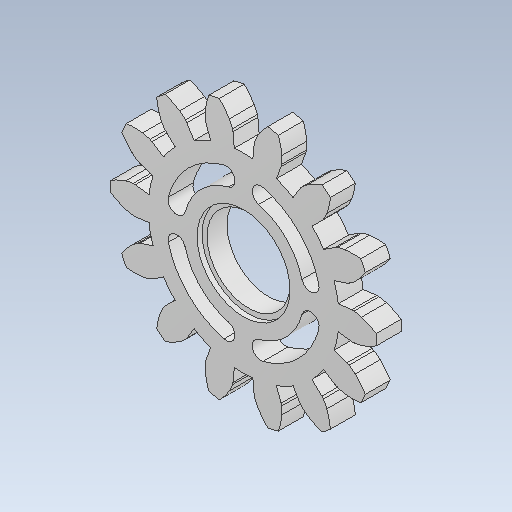
# Autodesk Inventor part: ｍ2歯数14ギアd10
Saved by Autodesk Inventor 2020.2 (Build 242310000, 310)
## iProperties
Created: 2020-03-09
Part Number: ｍ2歯数14ギアd10
Material: アルミニウム 2014-T4
Document SubType Name: Modeling
Designer: aoyam
Density: 2.8 g/cm^3
Appearance: サテン
Mass: 4.28588 g
Surface Area: 16.7705 cm^2
Volume: 1.53067 cm^3
Author: aoyam
Autodesk Inventor part; units mm, degrees
ref_plane "YZ Plane" through (0, 0, 0) normal (1, 0, 0) x (0, 1, 0)
ref_plane "XZ Plane" through (0, 0, 0) normal (0, 1, 0) x (-1, 0, 0)
ref_plane "XY Plane" through (0, 0, 0) normal (0, 0, 1) x (1, 0, 0)
sketch "スケッチ1" plane through (0, 0, 0) normal (0, 0, 1) x (1, 0, 0)
  arc A0 (3.027306, 14.807993) -> (2.963603, 14.540405) centre (4.457622, 14.32611) ccw
  arc A1 (3.408783, 15.648143) -> (3.027306, 14.807993) centre (7.00507, 13.50854) ccw
  arc A2 (4.613453, 17.176768) -> (3.408783, 15.648143) centre (9.745262, 11.893521) ccw
  arc A3 (0.407664, 14.540405) -> (0.343961, 14.807993) centre (-1.086355, 14.32611) ccw
  arc A4 (0.343961, 14.807993) -> (-0.037516, 15.648143) centre (-3.633803, 13.50854) ccw
  arc A5 (-0.037516, 15.648143) -> (-1.242186, 17.176768) centre (-6.373995, 11.893521) ccw
  arc A6 (2.802766, 12.892539) -> (0.568501, 12.892539) centre (1.685634, 1.446928) ccw
  arc A7 (-1.242186, 17.176768) -> (-2.501414, 16.889357) centre (1.685634, 1.446928) ccw
  line L0 (2.802766, 12.892539) -> (2.963603, 14.540405)
  line L1 (0.568501, 12.892539) -> (0.407664, 14.540405)
  arc A8 (-6.028546, 13.494134) -> (-7.777163, 14.34869) centre (-10.108448, 7.362041) ccw
  arc A9 (-7.777163, 14.34869) -> (-8.786985, 13.543384) centre (1.685634, 1.446928) ccw
  arc A10 (-5.320321, 12.902702) -> (-6.028546, 13.494134) centre (-8.340351, 10.006048) ccw
  arc A11 (-5.146824, 12.689253) -> (-5.320321, 12.902702) centre (-6.39991, 11.847949) ccw
  line L2 (-4.286932, 11.274361) -> (-5.146824, 12.689253)
  arc A12 (-2.90271, 14.066962) -> (-2.844002, 13.798233) centre (-1.404959, 14.253391) ccw
  arc A13 (-2.923539, 14.989427) -> (-2.90271, 14.066962) centre (1.244943, 14.622082) ccw
  arc A14 (-2.501414, 16.889357) -> (-2.923539, 14.989427) centre (4.414501, 14.355925) ccw
  line L3 (-2.27393, 12.243772) -> (-2.844002, 13.798233)
  arc A15 (-2.27393, 12.243772) -> (-4.286932, 11.274361) centre (1.685634, 1.446928) ccw
  arc A16 (-10.491689, 8.954028) -> (-12.437917, 8.965261) centre (-11.506938, 1.659001) ccw
  arc A17 (-12.437917, 8.965261) -> (-12.998325, 7.80156) centre (1.685634, 1.446928) ccw
  arc A18 (-9.596987, 8.728454) -> (-10.491689, 8.954028) centre (-11.061129, 4.808317) ccw
  arc A19 (-9.34806, 8.61142) -> (-9.596987, 8.728454) centre (-10.112023, 7.309739) ccw
  line L4 (-7.959426, 7.70974) -> (-9.34806, 8.61142)
  arc A20 (-7.923949, 10.826378) -> (-7.754458, 10.609734) centre (-6.65541, 11.644194) ccw
  arc A21 (-8.342958, 11.648453) -> (-7.923949, 10.826378) centre (-4.4279, 13.126123) ccw
  arc A22 (-8.786985, 13.543384) -> (-8.342958, 11.648453) centre (-1.456746, 14.261543) ccw
  line L5 (-6.566385, 9.456558) -> (-7.754458, 10.609734)
  arc A23 (-6.566385, 9.456558) -> (-7.959426, 7.70974) centre (1.685634, 1.446928) ccw
  arc A24 (-12.542964, 2.927049) -> (-14.301328, 2.092733) centre (-10.292478, -4.086043) ccw
  arc A25 (-14.301328, 2.092733) -> (-14.301328, 0.801122) centre (1.685634, 1.446928) ccw
  arc A26 (-11.638992, 3.11201) -> (-12.542964, 2.927049) centre (-11.257255, -1.055178) ccw
  arc A27 (-11.363938, 3.114572) -> (-11.638992, 3.11201) centre (-11.487466, 1.610326) ccw
  line L6 (-9.721598, 2.904692) -> (-11.363938, 3.114572)
  arc A28 (-11.041892, 5.728079) -> (-10.795188, 5.606429) centre (-10.253815, 7.015304) ccw
  arc A29 (-11.776091, 6.286941) -> (-11.041892, 5.728079) centre (-8.889883, 9.316956) ccw
  arc A30 (-12.998325, 7.80156) -> (-11.776091, 6.286941) centre (-6.705606, 11.62907) ccw
  line L7 (-9.224427, 5.082939) -> (-10.795188, 5.606429)
  arc A31 (-9.224427, 5.082939) -> (-9.721598, 2.904692) centre (1.685634, 1.446928) ccw
  arc A32 (-11.776091, -3.393086) -> (-12.998325, -4.907705) centre (-6.705606, -8.735215) ccw
  arc A33 (-12.998325, -4.907705) -> (-12.437917, -6.071406) centre (1.685634, 1.446928) ccw
  arc A34 (-11.041892, -2.834223) -> (-11.776091, -3.393086) centre (-8.889883, -6.423101) ccw
  arc A35 (-10.795188, -2.712574) -> (-11.041892, -2.834223) centre (-10.253815, -4.121449) ccw
  line L8 (-9.224427, -2.189084) -> (-10.795188, -2.712574)
  arc A36 (-11.638992, -0.218155) -> (-11.363938, -0.220717) centre (-11.487466, 1.283529) ccw
  arc A37 (-12.542964, -0.033194) -> (-11.638992, -0.218155) centre (-11.257255, 3.949033) ccw
  arc A38 (-14.301328, 0.801122) -> (-12.542964, -0.033194) centre (-10.292478, 6.979898) ccw
  line L9 (-9.721598, -0.010837) -> (-11.363938, -0.220717)
  arc A39 (-9.721598, -0.010837) -> (-9.224427, -2.189084) centre (1.685634, 1.446928) ccw
  arc A40 (-8.342958, -8.754598) -> (-8.786985, -10.649529) centre (-1.456746, -11.367688) ccw
  arc A41 (-8.786985, -10.649529) -> (-7.777163, -11.454835) centre (1.685634, 1.446928) ccw
  arc A42 (-7.923949, -7.932523) -> (-8.342958, -8.754598) centre (-4.4279, -10.232268) ccw
  arc A43 (-7.754458, -7.715879) -> (-7.923949, -7.932523) centre (-6.65541, -8.750339) ccw
  line L10 (-6.566385, -6.562703) -> (-7.754458, -7.715879)
  arc A44 (-9.596987, -5.834599) -> (-9.34806, -5.717565) centre (-10.112023, -4.415883) ccw
  arc A45 (-10.491689, -6.060173) -> (-9.596987, -5.834599) centre (-11.061129, -1.914462) ccw
  arc A46 (-12.437917, -6.071406) -> (-10.491689, -6.060173) centre (-11.506938, 1.234854) ccw
  line L11 (-7.959426, -4.815885) -> (-9.34806, -5.717565)
  arc A47 (-7.959426, -4.815885) -> (-6.566385, -6.562703) centre (1.685634, 1.446928) ccw
  arc A48 (-2.923539, -12.095572) -> (-2.501414, -13.995502) centre (4.414501, -11.462069) ccw
  arc A49 (-2.501414, -13.995502) -> (-1.242186, -14.282913) centre (1.685634, 1.446928) ccw
  arc A50 (-2.90271, -11.173107) -> (-2.923539, -12.095572) centre (1.244943, -11.728227) ccw
  arc A51 (-2.844002, -10.904378) -> (-2.90271, -11.173107) centre (-1.404959, -11.359536) ccw
  line L12 (-2.27393, -9.349917) -> (-2.844002, -10.904378)
  arc A52 (-5.320321, -10.008847) -> (-5.146824, -9.795398) centre (-6.39991, -8.954094) ccw
  arc A53 (-6.028546, -10.600279) -> (-5.320321, -10.008847) centre (-8.340351, -7.112193) ccw
  arc A54 (-7.777163, -11.454835) -> (-6.028546, -10.600279) centre (-10.108448, -4.468186) ccw
  line L13 (-4.286932, -8.380506) -> (-5.146824, -9.795398)
  arc A55 (-4.286932, -8.380506) -> (-2.27393, -9.349917) centre (1.685634, 1.446928) ccw
  arc A56 (3.408783, -12.754288) -> (4.613453, -14.282913) centre (9.745262, -8.999666) ccw
  arc A57 (4.613453, -14.282913) -> (5.872681, -13.995502) centre (1.685634, 1.446928) ccw
  arc A58 (3.027306, -11.914138) -> (3.408783, -12.754288) centre (7.00507, -10.614685) ccw
  arc A59 (2.963603, -11.64655) -> (3.027306, -11.914138) centre (4.457622, -11.432255) ccw
  line L14 (2.802766, -9.998684) -> (2.963603, -11.64655)
  arc A60 (0.343961, -11.914138) -> (0.407664, -11.64655) centre (-1.086355, -11.432255) ccw
  arc A61 (-0.037516, -12.754288) -> (0.343961, -11.914138) centre (-3.633803, -10.614685) ccw
  arc A62 (-1.242186, -14.282913) -> (-0.037516, -12.754288) centre (-6.373995, -8.999666) ccw
  line L15 (0.568501, -9.998684) -> (0.407664, -11.64655)
  arc A63 (0.568501, -9.998684) -> (2.802766, -9.998684) centre (1.685634, 1.446928) ccw
  arc A64 (9.399814, -10.600279) -> (11.14843, -11.454835) centre (13.479715, -4.468186) ccw
  arc A65 (11.14843, -11.454835) -> (12.158252, -10.649529) centre (1.685634, 1.446928) ccw
  arc A66 (8.691588, -10.008847) -> (9.399814, -10.600279) centre (11.711618, -7.112193) ccw
  arc A67 (8.518091, -9.795398) -> (8.691588, -10.008847) centre (9.771177, -8.954094) ccw
  line L16 (7.658199, -8.380506) -> (8.518091, -9.795398)
  arc A68 (6.273977, -11.173107) -> (6.21527, -10.904378) centre (4.776226, -11.359536) ccw
  arc A69 (6.294806, -12.095572) -> (6.273977, -11.173107) centre (2.126324, -11.728227) ccw
  arc A70 (5.872681, -13.995502) -> (6.294806, -12.095572) centre (-1.043234, -11.462069) ccw
  line L17 (5.645197, -9.349917) -> (6.21527, -10.904378)
  arc A71 (5.645197, -9.349917) -> (7.658199, -8.380506) centre (1.685634, 1.446928) ccw
  arc A72 (13.862957, -6.060173) -> (15.809184, -6.071406) centre (14.878205, 1.234854) ccw
  arc A73 (15.809184, -6.071406) -> (16.369593, -4.907705) centre (1.685634, 1.446928) ccw
  arc A74 (12.968255, -5.834599) -> (13.862957, -6.060173) centre (14.432396, -1.914462) ccw
  arc A75 (12.719327, -5.717565) -> (12.968255, -5.834599) centre (13.48329, -4.415883) ccw
  line L18 (11.330693, -4.815885) -> (12.719327, -5.717565)
  arc A76 (11.295216, -7.932523) -> (11.125725, -7.715879) centre (10.026677, -8.750339) ccw
  arc A77 (11.714225, -8.754598) -> (11.295216, -7.932523) centre (7.799167, -10.232268) ccw
  arc A78 (12.158252, -10.649529) -> (11.714225, -8.754598) centre (4.828013, -11.367688) ccw
  line L19 (9.937652, -6.562703) -> (11.125725, -7.715879)
  arc A79 (9.937652, -6.562703) -> (11.330693, -4.815885) centre (1.685634, 1.446928) ccw
  arc A80 (15.914231, -0.033194) -> (17.672595, 0.801122) centre (13.663745, 6.979898) ccw
  arc A81 (17.672595, 0.801122) -> (17.672595, 2.092733) centre (1.685634, 1.446928) ccw
  arc A82 (15.01026, -0.218155) -> (15.914231, -0.033194) centre (14.628522, 3.949033) ccw
  arc A83 (14.735205, -0.220717) -> (15.01026, -0.218155) centre (14.858733, 1.283529) ccw
  line L20 (13.092865, -0.010837) -> (14.735205, -0.220717)
  arc A84 (14.413159, -2.834223) -> (14.166455, -2.712574) centre (13.625082, -4.121449) ccw
  arc A85 (15.147358, -3.393086) -> (14.413159, -2.834223) centre (12.26115, -6.423101) ccw
  arc A86 (16.369593, -4.907705) -> (15.147358, -3.393086) centre (10.076873, -8.735215) ccw
  line L21 (12.595694, -2.189084) -> (14.166455, -2.712574)
  arc A87 (12.595694, -2.189084) -> (13.092865, -0.010837) centre (1.685634, 1.446928) ccw
  arc A88 (15.147358, 6.286941) -> (16.369593, 7.80156) centre (10.076873, 11.62907) ccw
  arc A89 (16.369593, 7.80156) -> (15.809184, 8.965261) centre (1.685634, 1.446928) ccw
  arc A90 (14.413159, 5.728079) -> (15.147358, 6.286941) centre (12.26115, 9.316956) ccw
  arc A91 (14.166455, 5.606429) -> (14.413159, 5.728079) centre (13.625082, 7.015304) ccw
  line L22 (12.595694, 5.082939) -> (14.166455, 5.606429)
  arc A92 (15.01026, 3.11201) -> (14.735205, 3.114572) centre (14.858733, 1.610326) ccw
  arc A93 (15.914231, 2.927049) -> (15.01026, 3.11201) centre (14.628522, -1.055178) ccw
  arc A94 (17.672595, 2.092733) -> (15.914231, 2.927049) centre (13.663745, -4.086043) ccw
  line L23 (13.092865, 2.904692) -> (14.735205, 3.114572)
  arc A95 (13.092865, 2.904692) -> (12.595694, 5.082939) centre (1.685634, 1.446928) ccw
  arc A96 (11.714225, 11.648453) -> (12.158252, 13.543384) centre (4.828013, 14.261543) ccw
  arc A97 (12.158252, 13.543384) -> (11.14843, 14.34869) centre (1.685634, 1.446928) ccw
  arc A98 (11.295216, 10.826378) -> (11.714225, 11.648453) centre (7.799167, 13.126123) ccw
  arc A99 (11.125725, 10.609734) -> (11.295216, 10.826378) centre (10.026677, 11.644194) ccw
  line L24 (9.937652, 9.456558) -> (11.125725, 10.609734)
  arc A100 (12.968255, 8.728454) -> (12.719327, 8.61142) centre (13.48329, 7.309739) ccw
  arc A101 (13.862957, 8.954028) -> (12.968255, 8.728454) centre (14.432396, 4.808317) ccw
  arc A102 (15.809184, 8.965261) -> (13.862957, 8.954028) centre (14.878205, 1.659001) ccw
  line L25 (11.330693, 7.70974) -> (12.719327, 8.61142)
  arc A103 (11.330693, 7.70974) -> (9.937652, 9.456558) centre (1.685634, 1.446928) ccw
  arc A104 (6.294806, 14.989427) -> (5.872681, 16.889357) centre (-1.043234, 14.355925) ccw
  arc A105 (5.872681, 16.889357) -> (4.613453, 17.176768) centre (1.685634, 1.446928) ccw
  arc A106 (6.273977, 14.066962) -> (6.294806, 14.989427) centre (2.126324, 14.622082) ccw
  arc A107 (6.21527, 13.798233) -> (6.273977, 14.066962) centre (4.776226, 14.253391) ccw
  line L26 (5.645197, 12.243772) -> (6.21527, 13.798233)
  arc A108 (8.691588, 12.902702) -> (8.518091, 12.689253) centre (9.771177, 11.847949) ccw
  arc A109 (9.399814, 13.494134) -> (8.691588, 12.902702) centre (11.711618, 10.006048) ccw
  arc A110 (11.14843, 14.34869) -> (9.399814, 13.494134) centre (13.479715, 7.362041) ccw
  line L27 (7.658199, 11.274361) -> (8.518091, 12.689253)
  arc A111 (7.658199, 11.274361) -> (5.645197, 12.243772) centre (1.685634, 1.446928) ccw
  circle A112 centre (1.685634, 1.446928) radius 5
  circle A113 centre (1.685634, 1.446928) radius 11.5
  circle A114 centre (1.685634, 1.446928) radius 9.375343
  circle A115 centre (1.685634, 1.446928) radius 7.275343
  line L28 (6.685634, 1.446928) -> (-7.68971, 1.446928)
  circle A116 centre (-6.373995, 3.533487) radius 1.05
  circle A117 centre (-6.373995, -0.639632) radius 1.05
  circle A118 centre (-0.400926, -6.612701) radius 1.05
  circle A119 centre (3.772193, -6.612701) radius 1.05
  circle A120 centre (9.745262, -0.639632) radius 1.05
  circle A121 centre (9.745262, 3.533487) radius 1.05
  circle A122 centre (3.772193, 9.506556) radius 1.05
  circle A123 centre (-0.400926, 9.506556) radius 1.05
  point P0 (0, 0)
  point P1 (6.21527, 13.798233)
  point P2 (6.273977, 14.066962)
  point P3 (6.294806, 14.989427)
  point P4 (5.872681, 16.889357)
  point P5 (4.613453, 17.176768)
  point P6 (3.408783, 15.648143)
  point P7 (3.027306, 14.807993)
  point P8 (0.343961, 14.807993)
  point P9 (-0.037516, 15.648143)
  point P10 (-1.242186, 17.176768)
  point P11 (-2.501414, 16.889357)
  point P12 (-2.923539, 14.989427)
  point P13 (-2.90271, 14.066962)
  point P14 (-2.844002, 13.798233)
  point P15 (-2.27393, 12.243772)
  point P16 (-4.286932, 11.274361)
  point P17 (-5.146824, 12.689253)
  point P18 (-5.320321, 12.902702)
  point P19 (-6.028546, 13.494134)
  point P20 (-7.777163, 14.34869)
  point P21 (-8.786985, 13.543384)
  point P22 (-8.342958, 11.648453)
  point P23 (-7.754458, 10.609734)
  point P24 (-6.566385, 9.456558)
  point P25 (-7.959426, 7.70974)
  point P26 (-9.34806, 8.61142)
  point P27 (-9.596987, 8.728454)
  point P28 (-10.491689, 8.954028)
  point P29 (-12.437917, 8.965261)
  point P30 (-12.998325, 7.80156)
  point P31 (-11.776091, 6.286941)
  point P32 (-11.041892, 5.728079)
  point P33 (-10.795188, 5.606429)
  point P34 (-11.363938, 3.114572)
  point P35 (-11.638992, 3.11201)
  point P36 (-12.542964, 2.927049)
  point P37 (-14.301328, 2.092733)
  point P38 (-14.301328, 0.801122)
  point P39 (-12.542964, -0.033194)
  point P40 (-11.638992, -0.218155)
  point P41 (-11.363938, -0.220717)
  point P42 (-9.721598, -0.010837)
  point P43 (-10.795188, -2.712574)
  point P44 (-11.041892, -2.834223)
  point P45 (-11.776091, -3.393086)
  point P46 (-12.998325, -4.907705)
  point P47 (-12.437917, -6.071406)
  point P48 (-10.491689, -6.060173)
  point P49 (-9.596987, -5.834599)
  point P50 (-9.34806, -5.717565)
  point P51 (-7.923949, -7.932523)
  point P52 (-8.342958, -8.754598)
  point P53 (-8.786985, -10.649529)
  point P54 (-7.777163, -11.454835)
  point P55 (-6.028546, -10.600279)
  point P56 (-5.320321, -10.008847)
  point P57 (-5.146824, -9.795398)
  point P58 (-4.286932, -8.380506)
  point P59 (-2.844002, -10.904378)
  point P60 (-2.90271, -11.173107)
  point P61 (-2.923539, -12.095572)
  point P62 (-2.501414, -13.995502)
  point P63 (-1.242186, -14.282913)
  point P64 (-0.037516, -12.754288)
  point P65 (0.343961, -11.914138)
  point P66 (0.568501, -9.998684)
  point P67 (2.802766, -9.998684)
  point P68 (3.027306, -11.914138)
  point P69 (3.408783, -12.754288)
  point P70 (4.613453, -14.282913)
  point P71 (5.872681, -13.995502)
  point P72 (6.294806, -12.095572)
  point P73 (6.273977, -11.173107)
  point P74 (5.645197, -9.349917)
  point P75 (7.658199, -8.380506)
  point P76 (8.691588, -10.008847)
  point P77 (9.399814, -10.600279)
  point P78 (11.14843, -11.454835)
  point P79 (12.158252, -10.649529)
  point P80 (11.295216, -7.932523)
  point P81 (11.125725, -7.715879)
  point P82 (12.719327, -5.717565)
  point P83 (12.968255, -5.834599)
  point P84 (13.862957, -6.060173)
  point P85 (15.809184, -6.071406)
  point P86 (16.369593, -4.907705)
  point P87 (15.147358, -3.393086)
  point P88 (14.413159, -2.834223)
  point P89 (14.166455, -2.712574)
  point P90 (14.735205, -0.220717)
  point P91 (15.01026, -0.218155)
  point P92 (15.914231, -0.033194)
  point P93 (17.672595, 0.801122)
  point P94 (17.672595, 2.092733)
  point P95 (15.914231, 2.927049)
  point P96 (15.01026, 3.11201)
  point P97 (13.092865, 2.904692)
  point P98 (12.595694, 5.082939)
  point P99 (14.413159, 5.728079)
  point P100 (15.147358, 6.286941)
  point P101 (16.369593, 7.80156)
  point P102 (15.809184, 8.965261)
  point P103 (13.862957, 8.954028)
  point P104 (12.968255, 8.728454)
  point P105 (11.330693, 7.70974)
  point P106 (9.937652, 9.456558)
  point P107 (11.295216, 10.826378)
  point P108 (11.714225, 11.648453)
  point P109 (12.158252, 13.543384)
  point P110 (11.14843, 14.34869)
  point P111 (9.399814, 13.494134)
  point P112 (8.518091, 12.689253)
  point P113 (-5.357507, 3.270328)
  point P114 (-7.390483, 3.796646)
  point P115 (-0.664085, 10.523044)
  point P116 (-0.137767, 8.490068)
  point P117 (4.035352, -7.629189)
  point P118 (3.509034, -5.596213)
  point P119 (8.728774, -0.376473)
  point P120 (10.76175, -0.902791)
  point P121 (10.76175, 3.796646)
  point P122 (8.728774, 3.270328)
  point P123 (3.509034, 8.490068)
  point P124 (4.035352, 10.523044)
  point P125 (-7.390483, -0.902791)
  point P126 (-5.357507, -0.376473)
  point P127 (-0.137767, -5.596213)
  point P128 (-0.664085, -7.629189)
  dimension "d4" = 10
  dimension "d2" = 360
  dimension "d21" = 2.12466
  dimension "d22" = 2.27534
  dimension "d24" = 2.1
  dimension "d27" = 360
  constraints: 224 point on circle, 122 centre point, 58 end point, 3 coincident, 1 horizontal alignment, 1 point on line, 1 symmetric about line, 1 tangent, 594 other
  measures "d24" diameter of A116
sketch "スケッチ1 outline for 押し出し1" plane through (0, 0, 0) normal (0, 0, 1) x (1, 0, 0)
  arc A0 (11.295216, -7.932523) -> (11.125725, -7.715879) centre (10.026677, -8.750339) ccw
  arc A1 (11.714225, -8.754598) -> (11.295216, -7.932523) centre (7.799167, -10.232268) ccw
  line L0 (11.125725, -7.715879) -> (9.937652, -6.562703)
  arc A2 (12.158252, -10.649529) -> (11.714225, -8.754598) centre (4.828013, -11.367688) ccw
  arc A3 (9.937652, -6.562703) -> (11.330693, -4.815885) centre (1.685634, 1.446928) ccw
  arc A4 (11.14843, -11.454835) -> (12.158252, -10.649529) centre (1.685634, 1.446928) ccw
  line L1 (11.330693, -4.815885) -> (12.719327, -5.717565)
  arc A5 (9.399814, -10.600279) -> (11.14843, -11.454835) centre (13.479715, -4.468186) ccw
  arc A6 (12.719327, -5.717565) -> (12.968255, -5.834599) centre (13.48329, -4.415883) ccw
  arc A7 (8.691588, -10.008847) -> (9.399814, -10.600279) centre (11.711618, -7.112193) ccw
  arc A8 (12.968255, -5.834599) -> (13.862957, -6.060173) centre (14.432396, -1.914462) ccw
  arc A9 (8.518091, -9.795398) -> (8.691588, -10.008847) centre (9.771177, -8.954094) ccw
  arc A10 (13.862957, -6.060173) -> (15.809184, -6.071406) centre (14.878205, 1.234854) ccw
  line L2 (7.658199, -8.380506) -> (8.518091, -9.795398)
  arc A11 (15.809184, -6.071406) -> (16.369593, -4.907705) centre (1.685634, 1.446928) ccw
  arc A12 (5.645197, -9.349917) -> (7.658199, -8.380506) centre (1.685634, 1.446928) ccw
  arc A13 (16.369593, -4.907705) -> (15.147358, -3.393086) centre (10.076873, -8.735215) ccw
  line L3 (6.21527, -10.904378) -> (5.645197, -9.349917)
  arc A14 (15.147358, -3.393086) -> (14.413159, -2.834223) centre (12.26115, -6.423101) ccw
  arc A15 (6.273977, -11.173107) -> (6.21527, -10.904378) centre (4.776226, -11.359536) ccw
  arc A16 (14.413159, -2.834223) -> (14.166455, -2.712574) centre (13.625082, -4.121449) ccw
  arc A17 (6.294806, -12.095572) -> (6.273977, -11.173107) centre (2.126324, -11.728227) ccw
  line L4 (14.166455, -2.712574) -> (12.595694, -2.189084)
  arc A18 (5.872681, -13.995502) -> (6.294806, -12.095572) centre (-1.043234, -11.462069) ccw
  arc A19 (12.595694, -2.189084) -> (13.092865, -0.010837) centre (1.685634, 1.446928) ccw
  arc A20 (4.613453, -14.282913) -> (5.872681, -13.995502) centre (1.685634, 1.446928) ccw
  line L5 (13.092865, -0.010837) -> (14.735205, -0.220717)
  arc A21 (3.408783, -12.754288) -> (4.613453, -14.282913) centre (9.745262, -8.999666) ccw
  arc A22 (14.735205, -0.220717) -> (15.01026, -0.218155) centre (14.858733, 1.283529) ccw
  arc A23 (3.027306, -11.914138) -> (3.408783, -12.754288) centre (7.00507, -10.614685) ccw
  arc A24 (15.01026, -0.218155) -> (15.914231, -0.033194) centre (14.628522, 3.949033) ccw
  arc A25 (2.963603, -11.64655) -> (3.027306, -11.914138) centre (4.457622, -11.432255) ccw
  arc A26 (15.914231, -0.033194) -> (17.672595, 0.801122) centre (13.663745, 6.979898) ccw
  line L6 (2.802766, -9.998684) -> (2.963603, -11.64655)
  arc A27 (17.672595, 0.801122) -> (17.672595, 2.092733) centre (1.685634, 1.446928) ccw
  arc A28 (0.568501, -9.998684) -> (2.802766, -9.998684) centre (1.685634, 1.446928) ccw
  arc A29 (17.672595, 2.092733) -> (15.914231, 2.927049) centre (13.663745, -4.086043) ccw
  line L7 (0.407664, -11.64655) -> (0.568501, -9.998684)
  arc A30 (15.914231, 2.927049) -> (15.01026, 3.11201) centre (14.628522, -1.055178) ccw
  arc A31 (0.343961, -11.914138) -> (0.407664, -11.64655) centre (-1.086355, -11.432255) ccw
  arc A32 (15.01026, 3.11201) -> (14.735205, 3.114572) centre (14.858733, 1.610326) ccw
  arc A33 (-0.037516, -12.754288) -> (0.343961, -11.914138) centre (-3.633803, -10.614685) ccw
  line L8 (14.735205, 3.114572) -> (13.092865, 2.904692)
  arc A34 (-1.242186, -14.282913) -> (-0.037516, -12.754288) centre (-6.373995, -8.999666) ccw
  arc A35 (13.092865, 2.904692) -> (12.595694, 5.082939) centre (1.685634, 1.446928) ccw
  arc A36 (-2.501414, -13.995502) -> (-1.242186, -14.282913) centre (1.685634, 1.446928) ccw
  line L9 (12.595694, 5.082939) -> (14.166455, 5.606429)
  arc A37 (-2.923539, -12.095572) -> (-2.501414, -13.995502) centre (4.414501, -11.462069) ccw
  arc A38 (14.166455, 5.606429) -> (14.413159, 5.728079) centre (13.625082, 7.015304) ccw
  arc A39 (-2.90271, -11.173107) -> (-2.923539, -12.095572) centre (1.244943, -11.728227) ccw
  arc A40 (14.413159, 5.728079) -> (15.147358, 6.286941) centre (12.26115, 9.316956) ccw
  arc A41 (-2.844002, -10.904378) -> (-2.90271, -11.173107) centre (-1.404959, -11.359536) ccw
  arc A42 (15.147358, 6.286941) -> (16.369593, 7.80156) centre (10.076873, 11.62907) ccw
  line L10 (-2.27393, -9.349917) -> (-2.844002, -10.904378)
  arc A43 (16.369593, 7.80156) -> (15.809184, 8.965261) centre (1.685634, 1.446928) ccw
  arc A44 (-4.286932, -8.380506) -> (-2.27393, -9.349917) centre (1.685634, 1.446928) ccw
  arc A45 (15.809184, 8.965261) -> (13.862957, 8.954028) centre (14.878205, 1.659001) ccw
  line L11 (-5.146824, -9.795398) -> (-4.286932, -8.380506)
  arc A46 (13.862957, 8.954028) -> (12.968255, 8.728454) centre (14.432396, 4.808317) ccw
  arc A47 (-5.320321, -10.008847) -> (-5.146824, -9.795398) centre (-6.39991, -8.954094) ccw
  arc A48 (12.968255, 8.728454) -> (12.719327, 8.61142) centre (13.48329, 7.309739) ccw
  arc A49 (-6.028546, -10.600279) -> (-5.320321, -10.008847) centre (-8.340351, -7.112193) ccw
  line L12 (12.719327, 8.61142) -> (11.330693, 7.70974)
  arc A50 (-7.777163, -11.454835) -> (-6.028546, -10.600279) centre (-10.108448, -4.468186) ccw
  arc A51 (11.330693, 7.70974) -> (9.937652, 9.456558) centre (1.685634, 1.446928) ccw
  arc A52 (-8.786985, -10.649529) -> (-7.777163, -11.454835) centre (1.685634, 1.446928) ccw
  line L13 (9.937652, 9.456558) -> (11.125725, 10.609734)
  arc A53 (-8.342958, -8.754598) -> (-8.786985, -10.649529) centre (-1.456746, -11.367688) ccw
  arc A54 (11.125725, 10.609734) -> (11.295216, 10.826378) centre (10.026677, 11.644194) ccw
  arc A55 (-7.923949, -7.932523) -> (-8.342958, -8.754598) centre (-4.4279, -10.232268) ccw
  arc A56 (11.295216, 10.826378) -> (11.714225, 11.648453) centre (7.799167, 13.126123) ccw
  arc A57 (-7.754458, -7.715879) -> (-7.923949, -7.932523) centre (-6.65541, -8.750339) ccw
  arc A58 (11.714225, 11.648453) -> (12.158252, 13.543384) centre (4.828013, 14.261543) ccw
  line L14 (-6.566385, -6.562703) -> (-7.754458, -7.715879)
  arc A59 (12.158252, 13.543384) -> (11.14843, 14.34869) centre (1.685634, 1.446928) ccw
  arc A60 (-7.959426, -4.815885) -> (-6.566385, -6.562703) centre (1.685634, 1.446928) ccw
  arc A61 (11.14843, 14.34869) -> (9.399814, 13.494134) centre (13.479715, 7.362041) ccw
  line L15 (-9.34806, -5.717565) -> (-7.959426, -4.815885)
  arc A62 (9.399814, 13.494134) -> (8.691588, 12.902702) centre (11.711618, 10.006048) ccw
  arc A63 (-9.596987, -5.834599) -> (-9.34806, -5.717565) centre (-10.112023, -4.415883) ccw
  arc A64 (8.691588, 12.902702) -> (8.518091, 12.689253) centre (9.771177, 11.847949) ccw
  arc A65 (-10.491689, -6.060173) -> (-9.596987, -5.834599) centre (-11.061129, -1.914462) ccw
  line L16 (8.518091, 12.689253) -> (7.658199, 11.274361)
  arc A66 (-12.437917, -6.071406) -> (-10.491689, -6.060173) centre (-11.506938, 1.234854) ccw
  arc A67 (7.658199, 11.274361) -> (5.645197, 12.243772) centre (1.685634, 1.446928) ccw
  arc A68 (-12.998325, -4.907705) -> (-12.437917, -6.071406) centre (1.685634, 1.446928) ccw
  line L17 (5.645197, 12.243772) -> (6.21527, 13.798233)
  arc A69 (-11.776091, -3.393086) -> (-12.998325, -4.907705) centre (-6.705606, -8.735215) ccw
  arc A70 (6.21527, 13.798233) -> (6.273977, 14.066962) centre (4.776226, 14.253391) ccw
  arc A71 (-11.041892, -2.834223) -> (-11.776091, -3.393086) centre (-8.889883, -6.423101) ccw
  arc A72 (6.273977, 14.066962) -> (6.294806, 14.989427) centre (2.126324, 14.622082) ccw
  arc A73 (-10.795188, -2.712574) -> (-11.041892, -2.834223) centre (-10.253815, -4.121449) ccw
  arc A74 (6.294806, 14.989427) -> (5.872681, 16.889357) centre (-1.043234, 14.355925) ccw
  line L18 (-9.224427, -2.189084) -> (-10.795188, -2.712574)
  arc A75 (5.872681, 16.889357) -> (4.613453, 17.176768) centre (1.685634, 1.446928) ccw
  arc A76 (-9.721598, -0.010837) -> (-9.224427, -2.189084) centre (1.685634, 1.446928) ccw
  arc A77 (4.613453, 17.176768) -> (3.408783, 15.648143) centre (9.745262, 11.893521) ccw
  line L19 (-11.363938, -0.220717) -> (-9.721598, -0.010837)
  arc A78 (3.408783, 15.648143) -> (3.027306, 14.807993) centre (7.00507, 13.50854) ccw
  arc A79 (-11.638992, -0.218155) -> (-11.363938, -0.220717) centre (-11.487466, 1.283529) ccw
  arc A80 (3.027306, 14.807993) -> (2.963603, 14.540405) centre (4.457622, 14.32611) ccw
  arc A81 (-12.542964, -0.033194) -> (-11.638992, -0.218155) centre (-11.257255, 3.949033) ccw
  line L20 (2.963603, 14.540405) -> (2.802766, 12.892539)
  arc A82 (-14.301328, 0.801122) -> (-12.542964, -0.033194) centre (-10.292478, 6.979898) ccw
  arc A83 (2.802766, 12.892539) -> (0.568501, 12.892539) centre (1.685634, 1.446928) ccw
  arc A84 (-14.301328, 2.092733) -> (-14.301328, 0.801122) centre (1.685634, 1.446928) ccw
  line L21 (0.568501, 12.892539) -> (0.407664, 14.540405)
  arc A85 (-12.542964, 2.927049) -> (-14.301328, 2.092733) centre (-10.292478, -4.086043) ccw
  arc A86 (0.407664, 14.540405) -> (0.343961, 14.807993) centre (-1.086355, 14.32611) ccw
  arc A87 (-11.638992, 3.11201) -> (-12.542964, 2.927049) centre (-11.257255, -1.055178) ccw
  arc A88 (0.343961, 14.807993) -> (-0.037516, 15.648143) centre (-3.633803, 13.50854) ccw
  arc A89 (-11.363938, 3.114572) -> (-11.638992, 3.11201) centre (-11.487466, 1.610326) ccw
  arc A90 (-0.037516, 15.648143) -> (-1.242186, 17.176768) centre (-6.373995, 11.893521) ccw
  line L22 (-9.721598, 2.904692) -> (-11.363938, 3.114572)
  arc A91 (-1.242186, 17.176768) -> (-2.501414, 16.889357) centre (1.685634, 1.446928) ccw
  arc A92 (-9.224427, 5.082939) -> (-9.721598, 2.904692) centre (1.685634, 1.446928) ccw
  arc A93 (-2.501414, 16.889357) -> (-2.923539, 14.989427) centre (4.414501, 14.355925) ccw
  line L23 (-10.795188, 5.606429) -> (-9.224427, 5.082939)
  arc A94 (-2.923539, 14.989427) -> (-2.90271, 14.066962) centre (1.244943, 14.622082) ccw
  arc A95 (-11.041892, 5.728079) -> (-10.795188, 5.606429) centre (-10.253815, 7.015304) ccw
  arc A96 (-2.90271, 14.066962) -> (-2.844002, 13.798233) centre (-1.404959, 14.253391) ccw
  arc A97 (-11.776091, 6.286941) -> (-11.041892, 5.728079) centre (-8.889883, 9.316956) ccw
  line L24 (-2.844002, 13.798233) -> (-2.27393, 12.243772)
  arc A98 (-12.998325, 7.80156) -> (-11.776091, 6.286941) centre (-6.705606, 11.62907) ccw
  arc A99 (-2.27393, 12.243772) -> (-4.286932, 11.274361) centre (1.685634, 1.446928) ccw
  arc A100 (-12.437917, 8.965261) -> (-12.998325, 7.80156) centre (1.685634, 1.446928) ccw
  line L25 (-4.286932, 11.274361) -> (-5.146824, 12.689253)
  arc A101 (-10.491689, 8.954028) -> (-12.437917, 8.965261) centre (-11.506938, 1.659001) ccw
  arc A102 (-5.146824, 12.689253) -> (-5.320321, 12.902702) centre (-6.39991, 11.847949) ccw
  arc A103 (-9.596987, 8.728454) -> (-10.491689, 8.954028) centre (-11.061129, 4.808317) ccw
  arc A104 (-5.320321, 12.902702) -> (-6.028546, 13.494134) centre (-8.340351, 10.006048) ccw
  arc A105 (-9.34806, 8.61142) -> (-9.596987, 8.728454) centre (-10.112023, 7.309739) ccw
  arc A106 (-6.028546, 13.494134) -> (-7.777163, 14.34869) centre (-10.108448, 7.362041) ccw
  line L26 (-7.959426, 7.70974) -> (-9.34806, 8.61142)
  arc A107 (-7.777163, 14.34869) -> (-8.786985, 13.543384) centre (1.685634, 1.446928) ccw
  arc A108 (-6.566385, 9.456558) -> (-7.959426, 7.70974) centre (1.685634, 1.446928) ccw
  arc A109 (-8.786985, 13.543384) -> (-8.342958, 11.648453) centre (-1.456746, 14.261543) ccw
  line L27 (-7.754458, 10.609734) -> (-6.566385, 9.456558)
  arc A110 (-8.342958, 11.648453) -> (-7.923949, 10.826378) centre (-4.4279, 13.126123) ccw
  arc A111 (-7.923949, 10.826378) -> (-7.754458, 10.609734) centre (-6.65541, 11.644194) ccw
  arc A112 (-7.390483, -0.902791) -> (-5.357507, -0.376473) centre (-6.373995, -0.639632) cw
  arc A113 (-0.664085, -7.629189) -> (-7.390483, -0.902791) centre (1.685634, 1.446928) cw
  arc A114 (-0.137767, -5.596213) -> (-0.664085, -7.629189) centre (-0.400926, -6.612701) cw
  arc A115 (-5.357507, -0.376473) -> (-0.137767, -5.596213) centre (1.685634, 1.446928) ccw
  arc A116 (4.035352, -7.629189) -> (3.509034, -5.596213) centre (3.772193, -6.612701) cw
  arc A117 (10.76175, -0.902791) -> (4.035352, -7.629189) centre (1.685634, 1.446928) cw
  arc A118 (8.728774, -0.376473) -> (10.76175, -0.902791) centre (9.745262, -0.639632) cw
  arc A119 (3.509034, -5.596213) -> (8.728774, -0.376473) centre (1.685634, 1.446928) ccw
  circle A120 centre (1.685634, 1.446928) radius 5
  arc A121 (-5.357507, 3.270328) -> (-7.390483, 3.796646) centre (-6.373995, 3.533487) cw
  arc A122 (-0.137767, 8.490068) -> (-5.357507, 3.270328) centre (1.685634, 1.446928) ccw
  arc A123 (-0.664085, 10.523044) -> (-0.137767, 8.490068) centre (-0.400926, 9.506556) cw
  arc A124 (-7.390483, 3.796646) -> (-0.664085, 10.523044) centre (1.685634, 1.446928) cw
  arc A125 (10.76175, 3.796646) -> (8.728774, 3.270328) centre (9.745262, 3.533487) cw
  arc A126 (4.035352, 10.523044) -> (10.76175, 3.796646) centre (1.685634, 1.446928) cw
  arc A127 (3.509034, 8.490068) -> (4.035352, 10.523044) centre (3.772193, 9.506556) cw
  arc A128 (8.728774, 3.270328) -> (3.509034, 8.490068) centre (1.685634, 1.446928) ccw
extrude "押し出し1" add sketch "スケッチ1 outline for 押し出し1" along normal blind 3
sketch "スケッチ3" plane through (0, 0, 3) normal (0, 0, 1) x (1, 0, 0)
  circle A0 centre (1.685634, 1.446928) radius 5
  circle A1 centre (1.685634, 1.446928) radius 5.6
  point P0 (0, 0)
  dimension "d18" = 0.6
  constraints: 1 centre point
  measures "d18" radial gap between concentric circles of A0 A1
extrude "押し出し3" cut sketch "スケッチ3" against normal blind 0.6
